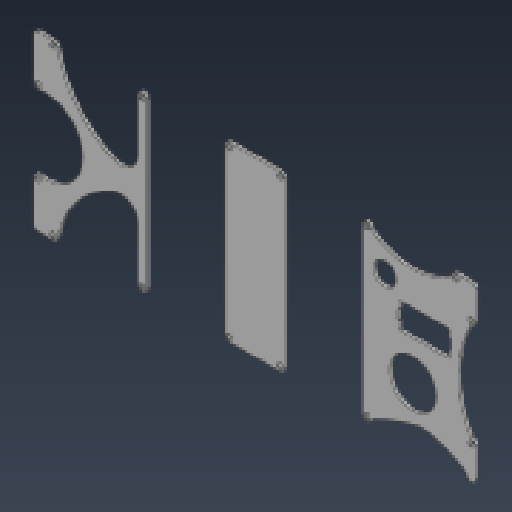
# Autodesk Inventor part: petg_skeleton_ceil
Saved by Autodesk Inventor 2023 (Build 270158000, 158)
## iProperties
Created: 2026-01-24
Part Number: petg_skeleton_ceil
Material: Generic
Document SubType Name: Modeling
Designer: szymo
Density: 1 g/cm^3
Appearance: Default
Author: szymo
Autodesk Inventor part; units mm, degrees
ref_plane "YZ Plane" through (0, 0, 0) normal (1, 0, 0) x (0, 1, 0)
ref_plane "XZ Plane" through (0, 0, 0) normal (0, 1, 0) x (-1, 0, 0)
ref_plane "XY Plane" through (0, 0, 0) normal (0, 0, 1) x (1, 0, 0)
ref_plane "Work Plane1" through (0, 0, 0) normal (0, 0, 1) x (1, 0, 0)
sketch "Sketch1" plane through (0, 0, 0) normal (0, 0, 1) x (1, 0, 0)
  circle A0 centre (116.5, 59.5) radius 1.5 projected
  circle A1 centre (-96.5, -91.5) radius 2.5 projected
  circle A2 centre (0, 91.5) radius 1.5 projected
  circle A3 centre (-96.5, 91.5) radius 1.5 projected
  circle A4 centre (0, -91.5) radius 1.5 projected
  circle A5 centre (99.5, 91.5) radius 1.5 projected
  circle A6 centre (116.5, -59.5) radius 1.5 projected
  line L0 (125, -100) -> (-125, -100) projected
  line L1 (125, 100) -> (125, -100) projected
  line L2 (-125, 100) -> (125, 100) projected
  line L3 (-125, 83) -> (-125, 100) projected
  line L4 (108, 83) -> (-125, 83) projected
  line L5 (108, -83) -> (108, 83) projected
  line L6 (-125, -83) -> (108, -83) projected
  line L7 (-125, -100) -> (-125, -83) projected
  circle A7 centre (-153.5, 91.5) radius 1.5 projected
  circle A8 centre (-250, -91.5) radius 1.5 projected
  circle A9 centre (-366.5, 45.75) radius 1.5 projected
  circle A10 centre (-349.5, -91.5) radius 1.5 projected
  circle A11 centre (-366.5, -45.75) radius 1.5 projected
  circle A12 centre (-349.5, 91.5) radius 1.5 projected
  circle A13 centre (-153.5, -91.5) radius 1.5 projected
  circle A14 centre (-250, 91.5) radius 1.5 projected
  line L8 (-375, 100) -> (-375, -100) projected
  line L9 (-375, -100) -> (-125, -100) projected
  line L10 (-125, -100) -> (-125, -83) projected
  line L11 (-125, -83) -> (-358, -83) projected
  line L12 (-358, -83) -> (-358, 83) projected
  line L13 (-358, 83) -> (-125, 83) projected
  line L14 (-125, 83) -> (-125, 100) projected
  line L15 (-125, 100) -> (-375, 100) projected
  circle A15 centre (-96.5, 91.5) radius 5
  circle A16 centre (-96.5, -91.5) radius 5
  circle A17 centre (0, -91.5) radius 5
  circle A18 centre (116.5, -59.5) radius 5
  circle A19 centre (116.5, 59.5) radius 5
  circle A20 centre (99.5, 91.5) radius 5
  circle A21 centre (0, 91.5) radius 5
  circle A22 centre (-153.5, 91.5) radius 5
  circle A23 centre (-153.5, -91.5) radius 5
  circle A24 centre (-250, -91.5) radius 5
  circle A25 centre (-349.5, -91.5) radius 5
  circle A26 centre (-366.5, -45.75) radius 5
  circle A27 centre (-366.5, 45.75) radius 5
  circle A28 centre (-349.5, 91.5) radius 5
  circle A29 centre (-250, 91.5) radius 5
  line L16 (-96.5, 96.5) -> (-153.5, 96.5)
  line L17 (-158.5, 91.5) -> (-158.5, -91.5)
  line L18 (-153.5, -96.5) -> (-96.5, -96.5)
  line L19 (-91.5, -91.5) -> (-91.5, 91.5)
  line L20 (-125, 83) -> (-125, -83) construction
  line L21 (-143.5, 64.5) -> (-143.5, -64.5)
  line L22 (-106.5, -64.5) -> (-106.5, 64.5)
  arc A30 (-106.5, 64.5) -> (-143.5, 64.5) centre (-125, 64.5) ccw
  arc A31 (-143.5, -64.5) -> (-106.5, -64.5) centre (-125, -64.5) ccw
  line L23 (-255, 91.5) -> (-255, -91.5)
  line L24 (-245, -91.5) -> (-245, 91.5)
  circle A32 centre (-366.5, 91.5) radius 5
  circle A33 centre (-366.5, -91.5) radius 5
  circle A34 centre (-366.5, 91.5) radius 0.5 projected
  circle A35 centre (-366.5, -91.5) radius 0.5 projected
  line L25 (-349.5, 96.5) -> (-366.5, 96.5)
  line L26 (-371.5, 91.5) -> (-371.5, 45.75)
  line L27 (-371.5, -45.75) -> (-371.5, -91.5)
  line L28 (-366.5, -96.5) -> (-349.5, -96.5)
  arc A36 (-255, -8) -> (-344.5, -91.5) centre (-241.6841, -111.9884) ccw
  arc A37 (-344.5, 91.5) -> (-255, 8) centre (-241.6841, 111.9884) ccw
  line L29 (-366.5, 45.75) -> (-366.5, 40.75)
  line L30 (-366.5, -45.75) -> (-366.5, -40.75)
  line L31 (-349.5, 91.5) -> (-344.5, 91.5)
  line L32 (-349.5, -91.5) -> (-344.5, -91.5)
  line L33 (-255, 0) -> (-316.3729, 0) construction
  arc A38 (-316.3729, 0) -> (-366.5, 40.75) centre (-358, 0) ccw
  arc A39 (-366.5, -40.75) -> (-316.3729, 0) centre (-358, 0) ccw
  circle A40 centre (-275, 33.9663) radius 20
  circle A41 centre (-275, -33.9663) radius 20
  circle A42 centre (-153.5, -91.5) radius 2.5 projected
  circle A43 centre (-96.5, 91.5) radius 2.5 projected
  circle A44 centre (-153.5, 91.5) radius 2.5 projected
  circle A45 centre (-250, 91.5) radius 2.5 projected
  circle A46 centre (-250, -91.5) radius 2.5 projected
  circle A47 centre (-349.5, -91.5) radius 2.5 projected
  circle A48 centre (-349.5, 91.5) radius 2.5 projected
  circle A49 centre (-366.5, 45.75) radius 2.5 projected
  circle A50 centre (-366.5, -45.75) radius 2.5 projected
  line L34 (-241.6841, 111.9884) -> (-241.6841, -111.9884) construction
  line L35 (-5, 91.5) -> (-5, -91.5)
  arc A51 (5, 91.5) -> (94.5, 91.5) centre (49.75, 149.1692) ccw
  arc A52 (116.5, -64.5) -> (5, -91.5) centre (116.5, -308.2269) ccw
  line L36 (116.5, -64.5) -> (116.5, -59.5)
  line L37 (5, -91.5) -> (0, -91.5)
  line L38 (99.5, 91.5) -> (94.5, 91.5)
  line L39 (0, 91.5) -> (5, 91.5)
  circle A53 centre (116.5, 91.5) radius 0.5 projected
  circle A54 centre (116.5, 91.5) radius 5
  line L40 (99.5, 96.5) -> (116.5, 96.5)
  line L41 (121.5, 91.5) -> (121.5, 59.5)
  arc A55 (116.5, 54.5) -> (116.5, -54.5) centre (210.2622, 0) ccw
  circle A56 centre (0, 91.5) radius 2.5 projected
  circle A57 centre (99.5, 91.5) radius 2.5 projected
  circle A58 centre (116.5, 59.5) radius 2.5 projected
  circle A59 centre (116.5, -59.5) radius 2.5 projected
  circle A60 centre (0, -91.5) radius 2.5 projected
  line L42 (116.5, -59.5) -> (116.5, -54.5)
  line L43 (116.5, 59.5) -> (116.5, 54.5)
  circle A61 centre (116.5, -91.5) radius 0.5 projected
  circle A62 centre (116.5, -91.5) radius 5
  line L44 (121.5, -59.5) -> (121.5, -91.5)
  arc A63 (111.5, -91.5) -> (59.1388, -71.3462) centre (51.2202, -170.0154) ccw
  line L45 (94.9469, 40.014) -> (94.9469, 9.014) projected
  arc A64 (93.9469, 8.014) -> (94.9469, 9.014) centre (93.9469, 9.014) ccw projected
  line L46 (93.9469, 8.014) -> (34.9469, 8.014) projected
  arc A65 (33.9469, 9.014) -> (34.9469, 8.014) centre (34.9469, 9.014) ccw projected
  line L47 (33.9469, 9.014) -> (33.9469, 40.014) projected
  arc A66 (34.9469, 41.014) -> (33.9469, 40.014) centre (34.9469, 40.014) ccw projected
  line L48 (34.9469, 41.014) -> (93.9469, 41.014) projected
  arc A67 (94.9469, 40.014) -> (93.9469, 41.014) centre (93.9469, 40.014) ccw projected
  line L49 (36.4469, 11.514) -> (36.4469, 37.514) projected
  arc A68 (36.4469, 11.514) -> (37.4469, 10.514) centre (37.4469, 11.514) ccw projected
  line L50 (91.4469, 10.514) -> (37.4469, 10.514) projected
  arc A69 (91.4469, 10.514) -> (92.4469, 11.514) centre (91.4469, 11.514) ccw projected
  line L51 (92.4469, 37.514) -> (92.4469, 11.514) projected
  arc A70 (92.4469, 37.514) -> (91.4469, 38.514) centre (91.4469, 37.514) ccw projected
  line L52 (37.4469, 38.514) -> (91.4469, 38.514) projected
  arc A71 (37.4469, 38.514) -> (36.4469, 37.514) centre (37.4469, 37.514) ccw projected
  line L53 (35.1469, 19.264) -> (35.1469, 29.764) projected
  line L54 (35.1469, 29.764) -> (36.4469, 29.764) projected
  line L55 (36.4469, 19.264) -> (36.4469, 29.764) projected
  line L56 (35.1469, 19.264) -> (36.4469, 19.264) projected
  line L57 (92.4469, 19.264) -> (92.4469, 29.764) projected
  line L58 (92.4469, 29.764) -> (93.7469, 29.764) projected
  line L59 (93.7469, 19.264) -> (93.7469, 29.764) projected
  line L60 (92.4469, 19.264) -> (93.7469, 19.264) projected
  arc A72 (36.2469, 11.514) -> (37.4469, 10.314) centre (37.4469, 11.514) ccw
  line L61 (36.2469, 11.514) -> (36.2469, 37.514)
  arc A73 (37.4469, 38.714) -> (36.2469, 37.514) centre (37.4469, 37.514) ccw
  line L62 (37.4469, 38.714) -> (91.4469, 38.714)
  arc A74 (92.6469, 37.514) -> (91.4469, 38.714) centre (91.4469, 37.514) ccw
  line L63 (92.6469, 37.514) -> (92.6469, 11.514)
  arc A75 (91.4469, 10.314) -> (92.6469, 11.514) centre (91.4469, 11.514) ccw
  line L64 (91.4469, 10.314) -> (37.4469, 10.314)
  line L65 (93.9469, 29.964) -> (92.2469, 29.964)
  line L66 (92.2469, 29.964) -> (92.2469, 19.064)
  line L67 (92.2469, 19.064) -> (93.9469, 19.064)
  line L68 (93.9469, 19.064) -> (93.9469, 29.964)
  line L69 (34.9469, 29.964) -> (34.9469, 19.064)
  line L70 (34.9469, 19.064) -> (36.6469, 19.064)
  line L71 (36.6469, 19.064) -> (36.6469, 29.964)
  line L72 (36.6469, 29.964) -> (34.9469, 29.964)
  circle A76 centre (51.2202, -33.9663) radius 26.1144
  circle A77 centre (20.1053, 56.1526) radius 12.5237
  point P0 (0, 0)
  point P1 (-125, 0)
  point P2 (-282.8541, -15.573)
  point P3 (-255, -33.9663)
  point P4 (-255, 33.9663)
  point P5 (-282.8541, 15.573)
  point P6 (-364.7041, 41.0837)
  point P7 (-282.8546, -15.5768)
  point P8 (-282.8549, 15.572)
  point P9 (-364.7041, -41.0837)
  point P10 (-358, -41.6271)
  point P11 (-342.4341, -83)
  point P12 (-342.4341, 83)
  point P13 (-358, 41.6271)
  point P14 (115.5177, -54.5974)
  point P15 (36.2469, 19.064)
  point P16 (36.2469, 29.964)
  point P17 (92.6469, 29.964)
  point P18 (92.6469, 19.064)
  dimension "d0" = 10
  dimension "d1" = 10
  dimension "d2" = 10
  dimension "d3" = 10
  dimension "d4" = 10
  dimension "d5" = 10
  dimension "d6" = 10
  dimension "d7" = 10
  dimension "d8" = 10
  dimension "d9" = 10
  dimension "d10" = 10
  dimension "d11" = 10
  dimension "d12" = 10
  dimension "d13" = 10
  dimension "d14" = 10
  dimension "d15" = 15
  dimension "d16" = 10
  dimension "d17" = 10
  dimension "d18" = 8
  dimension "d19" = 8
  dimension "d20" = 0
  dimension "d25" = 15
  dimension "d26" = 111.9883
  dimension "d27" = 111.9883
  dimension "d28" = 40
  dimension "d29" = 40
  dimension "d32" = 10
  dimension "d33" = 10
  dimension "d41" = 0.2
  dimension "d42" = 0.2
  dimension "d43" = 0.2
  constraints: 84 end point, 70 point on circle, 37 centre point, 25 tangent, 20 coincident, 7 horizontal, 7 point on line, 5 perpendicular, 5 vertical, 4 parallel, 2 midpoint, 17 other
  measures "d0" diameter of A15
  measures "d1" diameter of A16
  measures "d2" diameter of A17
  measures "d3" diameter of A18
  measures "d4" diameter of A19
  measures "d5" diameter of A20
  measures "d6" diameter of A21
  measures "d7" diameter of A22
  measures "d8" diameter of A23
  measures "d9" diameter of A24
  measures "d10" diameter of A25
  measures "d11" diameter of A26
  measures "d12" diameter of A27
  measures "d13" diameter of A28
  measures "d14" diameter of A29
  measures "d15" distance between parallel lines of L17 L21
  measures "d16" diameter of A32
  measures "d17" diameter of A33
  measures "d18" distance of A37.end L33.start
  measures "d19" distance of L33.start A36.start
  measures "d20" distance of A34.centre A32.centre
  measures "d26" distance from line of L34.start L33
  measures "d27" distance from line of L33 L34.end
  measures "d28" diameter of A40
  measures "d29" diameter of A41
  measures "d32" diameter of A54
  measures "d33" diameter of A62
  measures "d41" distance between parallel lines of L50 L64
  measures "d42" distance between parallel lines of L59 L68
  measures "d43" distance between parallel lines of L53 L69
extrude "Extrusion1" add sketch "Sketch1" along normal blind 3 contours L42 A18 L36 A59 | A59 L36 A18 L42 | A18 A52 L5 A55 | A18 L44 A62 A63 L6 L5 A52 | L5 A52 L6 L35 L4 A51 A55 | L5 L6 A63 A52 | A62 | L5 L4 A51 A20 L40 A54 L41 A19 A55 | A19 | A52 A17 L35 L6 | A17 | L4 L35 A21 A51 | A20 | A54 | L19 A16 L18 L7 L6 | L6 A31 L22 A30 L4 L19 | A21 | L7 L18 A23 L17 L11 | L11 L17 L13 A30 L21 A31 | A31 L21 A30 L22 | A16 | L4 L3 L16 A15 L19 | L13 L17 A22 L16 L3 | A15 | A23 | L24 A24 L23 L11 | L11 L23 L13 L24 | A24 | L13 L23 A29 L24 | A22 | A36 A25 L28 A33 L27 A26 A39 L12 L11 | L11 L12 A39 A38 L13 A37 L23 A36 | A41 A36 L23 | A29 | A25 | L13 L12 A38 A27 L26 A32 L25 A28 A37 | L23 A37 A40 | A28 | A39 A26 | A26 A39 | A33 | A38 A27 | A27 A38 | A32 | A34 | A35 | A53 | A61 | L45 A64 L46 A65 L47 A66 L48 A67
ref_plane "Work Plane2" through (-125, 0, 5) normal (0, 0, 1) x (1, 0, 0)
sketch "Sketch2" plane through (-125, 0, 5) normal (0, 0, 1) x (1, 0, 0)
  circle A0 centre (241.5, -59.5) radius 2.5 projected
  circle A1 centre (125, -91.5) radius 2.5 projected
  circle A2 centre (125, 91.5) radius 2.5 projected
  circle A3 centre (224.5, 91.5) radius 2.5 projected
  circle A4 centre (241.5, 59.5) radius 2.5 projected
  circle A5 centre (28.5, -91.5) radius 2.5 projected
  circle A6 centre (-28.5, -91.5) radius 2.5 projected
  circle A7 centre (-28.5, 91.5) radius 2.5 projected
  circle A8 centre (28.5, 91.5) radius 2.5 projected
  circle A9 centre (-125, -91.5) radius 2.5 projected
  circle A10 centre (-224.5, -91.5) radius 2.5 projected
  circle A11 centre (-224.5, 91.5) radius 2.5 projected
  circle A12 centre (-241.5, 45.75) radius 2.5 projected
  circle A13 centre (-241.5, -45.75) radius 2.5 projected
  circle A14 centre (-125, 91.5) radius 2.5 projected
  point P0 (125, 0)
hole "Hole1" at (116.5, -59.5, 5) at (0, -91.5, 5) at (0, 91.5, 5) at (99.5, 91.5, 5) at (116.5, 59.5, 5) at (-96.5, -91.5, 5) at (-153.5, -91.5, 5) at (-153.5, 91.5, 5) at (-96.5, 91.5, 5) at (-250, 91.5, 5) at (-349.5, 91.5, 5) at (-366.5, 45.75, 5) at (-366.5, -45.75, 5) at (-349.5, -91.5, 5) at (-250, -91.5, 5) direction (0, 0, -1) diameter 4.5 end through all countersink diameter 10 countersink angle 90 clearance for "Countersunk Flat Head Screw ISO 2009/7046" size "M4" standard "ISO"
equation "\"d19\" = d18"
body "Solid1"
